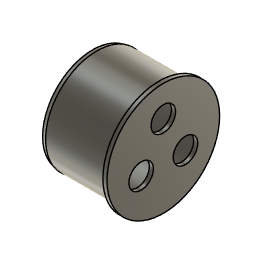
Stopfen DN50 mod v2 (Autodesk Fusion 360 design; units mm, degrees)
Autodesk Fusion 360 part; units mm, degrees
sketch "Skizze1" plane through (0, 0, 0) normal (0, 0, 1) x (1, 0, 0)
  line L0 (0, 0) -> (0, 27.5)
  line L1 (0, 27.5) -> (-2, 27.5)
  line L2 (-2, 27.5) -> (-2, 25)
  line L3 (-2, 25) -> (-32.5, 25)
  line L4 (-32.5, 25) -> (-34.5, 24.4641)
  line L5 (-34.5, 24.4641) -> (-34.5, 23)
  line L6 (-34.5, 23) -> (-2, 23)
  line L7 (-2, 23) -> (-2, 0)
  line L8 (-2, 0) -> (0, 0)
  dimension "d2" = 27.5
  dimension "d3" = 32.5
  dimension "d4" = 2
  dimension "d5" = 23
  dimension "d6" = 25
  dimension "d7" = 15
  dimension "d8" = 2
  constraint coincident L0.start L8.end
  constraint vertical L0
  constraint perpendicular L0 L1
  constraint perpendicular L1 L2
  constraint perpendicular L2 L3
  constraint perpendicular L3 L5
  constraint perpendicular L5 L6
  constraint perpendicular L6 L7
  constraint perpendicular L0 L8
  constraint collinear L2 L7
  measures "d2" distance of L0.start L0.end
  measures "d3" distance of L5.end L6.end
  measures "d4" distance of L0.end L1.end
  measures "d5" distance of L6.end L7.end
  measures "d6" distance of L3 L8
  measures "d7" angle of L3 L4
  measures "d8" distance of L3.end L5
revolve "Drehen1" add sketch "Skizze1" angle 360 about axis through (1.75, 0, 0) along (1, 0, 0)
sketch "Skizze3" plane through (0, 0, 0) normal (1, 0, 0) x (0, 1, 0)
  circle A0 centre (0, 0) radius 27.5
  circle A1 centre (-10.8253, -6.25) radius 6
  circle A2 centre (0, 12.5) radius 6
  circle A3 centre (10.8253, -6.25) radius 6
  line L0 (0, 0) -> (0, 27.5) construction
  line L1 (0, 0) -> (23.8157, -13.75) construction
  line L2 (0, 0) -> (-23.8157, -13.75) construction
  circle A4 centre (0, 0) radius 12.5 construction
  circle A5 centre (0, 0) radius 23
  circle A6 centre (0, 0) radius 23
  dimension "d9" = 120
  dimension "d10" = 120
  dimension "d11" = 12
  dimension "d12" = 25
  constraint coincident A0.centre L0.start
  constraint coincident A0 L0.end
  constraint vertical L0
  constraint coincident A0 L1.end
  constraint coincident A0 L2.end
  constraint coincident A2.centre L0
  constraint coincident A1.centre L2
  constraint coincident A3.centre L1
  constraint equal A2 A3
  constraint equal A1 A2
  constraint concentric A0 A4
  constraint coincident A2.centre A4
  constraint coincident A3.centre A4
  constraint coincident A1.centre A4
  measures "d9" angle of L0 L1
  measures "d10" angle of L0 L2
  measures "d11" diameter of A3
  measures "d12" diameter of A4
extrude "Extrusion1" cut sketch "Skizze3" against normal up to surface (2 mm away) contours A1 | A2 | A3
equation "d2 = ( 55 / 2 ) * 1 mm"
equation "d5 = ( 46 / 2 ) * 1 mm"
equation "d6 = ( 50 / 2 ) * 1 mm"
